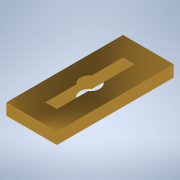
# Autodesk Inventor part: Acoplador
Saved by Autodesk Inventor 2020.1 (Build 241239000, 239)
## iProperties
Created: 2020-03-26
Part Number: Acoplador
Material: Brass
Document SubType Name: Modeling
Designer: Daniel
Density: 8.49 g/cm^3
Appearance: Brass - Polished
Author: Daniel
Autodesk Inventor part; units mm, degrees
ref_plane "YZ Plane" through (0, 0, 0) normal (1, 0, 0) x (0, 1, 0)
ref_plane "XZ Plane" through (0, 0, 0) normal (0, 1, 0) x (-1, 0, 0)
ref_plane "XY Plane" through (0, 0, 0) normal (0, 0, 1) x (1, 0, 0)
sketch "Sketch1" plane through (0, 0, 0) normal (0, 1, 0) x (-1, 0, 0)
  line L0 (-6.5, 15) -> (6.5, 15)
  line L1 (6.5, 15) -> (6.5, -15)
  line L2 (6.5, -15) -> (-6.5, -15)
  line L3 (-6.5, -15) -> (-6.5, 15)
  line L4 (-6.5, 15) -> (6.5, -15) construction
  line L5 (6.5, 15) -> (-6.5, -15) construction
  line L6 (-1.5, 10) -> (1.5, 10)
  line L7 (1.5, 10) -> (1.5, -10)
  line L8 (1.5, -10) -> (-1.5, -10)
  line L9 (-1.5, -10) -> (-1.5, 10)
  line L10 (-1.5, 10) -> (1.5, -10) construction
  line L11 (1.5, 10) -> (-1.5, -10) construction
  circle A0 centre (0, 0) radius 2.5
  point P0 (-1.5, -2)
  point P1 (-1.5, 2)
  point P2 (1.5, 2)
  point P3 (1.5, -2)
  dimension "d0" = 5
  dimension "d1" = 20
  dimension "d2" = 5
  dimension "d3" = 4
  dimension "d4" = 3
  constraints: 24 end point, 4 midpoint, 4 parallel, 2 horizontal, 2 perpendicular, 1 centre point, 1 coincident
  measures "d0" diameter of A0
  measures "d1" distance of L6.end L7.end
  measures "d2" distance between parallel lines of L2 L8
  measures "d3" distance edge to line of A0 L3
  measures "d4" distance of L7.end L8.end
extrude "Extrusion1" add sketch "Sketch1" along normal blind 3
body "Solid1"
